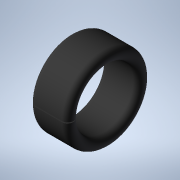
# Autodesk Inventor part: 8146543 ZBH-5-B
Saved by Autodesk Inventor 2021 (Build 250183000, 183)
## iProperties
Created: 2025-06-06
Part Number: 8146543 ZBH-5-B
Material: Generic
Catalog Web Link: www.cadenas.de
Description: ZBH-B-centring sleeve
Vendor: FESTO
Document SubType Name: Modeling
Designer: psAdmin
Manufacturer: FESTO
Mass: 1 g
Surface Area: 0.756677 cm^2
Volume: 0.0202619 cm^3
Density: 1 g/cm^3
Appearance: PSOLRGB-175-175-175
Category: PARTsolutions
Company: FESTO
Title: 8146543 ZBH-5-B
Author: Cadenas PARTsolutions
Comments: centring sleeve
PSOL_IDENT_0: {$CADENAS_DATA/23d-libs/festo/parts/z/zbh/zbh_b.prj},170 {VTYP=3D},{NB=8146543 ZBH-5-B},{LINA=814654
PSOL_IDENT_1: 3 ZBH-5-B},{NN=ZBH-B},{DATE=02.05.2024 17:22:15},{GEOMDATE=28.07.2023 08:56:26},{VERSION=},{LINEID=1
PSOL_IDENT_2: 00},{WBVAR=},{WBNUMERIC=}  {NB=8146543 ZBH-5-B},{LINA=8146543 ZBH-5-B},{KT=DUMMY},{TNR=8146543},{TYP=
PSOL_IDENT_3: ZBH-5-B},{B1=2.300},{D1=5.000},{D2=3.600},{CNSMASSEXACT=0.001},{GTIN=4052568610807}
NB: 8146543 ZBH-5-B
NN: ZBH-B
NT: centring sleeve
NBSYN: $TNR. $TYP.
LINA: 8146543 ZBH-5-B
CATALOG: Festo
TNR: 8146543
TYP: ZBH-5-B
B1: 2.3
D1: 5
D2: 3.6
CNSMASSEXACT: 0.001
GTIN: 4052568610807
SUPPLIER: FESTO
ARTICLENO: 8146543 ZBH-5-B
BOMINFO: 8146543 ZBH-5-B
CREATOR: CADENAS GmbH
Autodesk Inventor part; units mm, degrees
sketch "Sketch_3" plane through (0, 0, 0) normal (0, 0, 1) x (1, 0, 0)
  line L0 (2.3, 0) -> (0, 0)
  arc A0 (0.35, 2.5) -> (0.35, 1.8) centre (0.35, 2.15) ccw
  line L1 (0.35, 1.8) -> (1.95, 1.8)
  arc A1 (1.95, 1.8) -> (1.95, 2.5) centre (1.95, 2.15) ccw
  line L2 (1.95, 2.5) -> (0.35, 2.5)
  constraints: 6 end point, 4 point on circle, 2 centre point
revolve "Revolution1" add sketch "Sketch_3" angle 360 about axis through (2.3, 0, 0) along (-1, 0, 0)
sketch "Sketch_4" plane through (0, 0, 0) normal (1, 0, 0) x (0, 1, 0)
  arc A0 (0.0693, 3.4993) -> (-0.0693, 3.4993) centre (0, 0) ccw
  line L0 (-0.0693, 3.4993) -> (0, 1.5136)
  line L1 (0, 1.5136) -> (0.0693, 3.4993)
  constraints: 4 end point, 2 point on circle, 1 centre point
extrude "Extrusion1" cut sketch "Sketch_4" along normal blind 2.3
ref_plane "ANBAU_XY" through (0, 0, 0) normal (1, 0, 0) x (0, 0, -1)
ref_plane "ANBAU_YZ" through (0, 0, 0) normal (0, 0, -1) x (0, 1, 0)
ref_plane "ANBAU_ZX" through (0, 0, 0) normal (0, 1, 0) x (1, 0, 0)
ref_plane "insert_XY" through (0, 0, 0) normal (1, 0, 0) x (0, 0, -1)
ref_plane "insert_YZ" through (0, 0, 0) normal (0, 0, -1) x (0, 1, 0)
ref_plane "insert_ZX" through (0, 0, 0) normal (0, 1, 0) x (1, 0, 0)
ref_plane "schraube_punkt_XY" through (2.3, 0, 0) normal (1, 0, 0) x (0, 0, -1)
ref_plane "schraube_punkt_YZ" through (2.3, 0, 0) normal (0, 0, -1) x (0, 1, 0)
ref_plane "schraube_punkt_ZX" through (2.3, 0, 0) normal (0, 1, 0) x (1, 0, 0)
body "Solid1"
